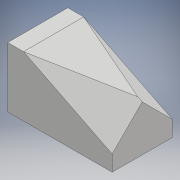
# Autodesk Inventor part: 6431
Saved by Autodesk Inventor 2017 (Build 210142000, 142)
## iProperties
Part Number: 6431
Material: 一般
Document SubType Name: Modeling
Designer: Brian
Density: 1 g/cm^3
Appearance: 預設
Mass: 79.3263 g
Surface Area: 112.179 cm^2
Volume: 79.3263 cm^3
Author: Brian
Autodesk Inventor part; units mm, degrees
ref_plane "YZ Plane" through (0, 0, 0) normal (1, 0, 0) x (0, 1, 0)
ref_plane "XZ Plane" through (0, 0, 0) normal (0, 1, 0) x (-1, 0, 0)
ref_plane "XY Plane" through (0, 0, 0) normal (0, 0, 1) x (1, 0, 0)
sketch "草圖1" plane through (0, 0, 0) normal (0, 1, 0) x (-1, 0, 0)
  line L0 (0, 0) -> (-66, 0)
  line L1 (-66, 0) -> (-66, -38)
  line L2 (-66, -38) -> (0, -38)
  line L3 (0, -38) -> (0, 0)
  dimension "d0" = 66
  dimension "d1" = 38
  constraints: 8 end point, 2 parallel, 1 horizontal, 1 perpendicular
  measures "d0" distance of L1.end L2.end
  measures "d1" distance of L2.end L0.start
extrude "擠出1" add sketch "草圖1" along normal mid plane 38
sketch "草圖2" plane through (0, 19, 0) normal (0, 1, 0) x (1, 0, 0)
  line L0 (0, 0) -> (66, 0) projected
  line L1 (10, 0) -> (66, 8)
  line L2 (66, 0) -> (66, 38) projected
  dimension "d4" = 10
  dimension "d5" = 30
  constraints: 2 end point, 2 point on line
  measures "d4" distance of L0.start L1.start
  measures "d5" distance of L2.end L1.end
extrude "擠出2" cut sketch "草圖2" against normal blind 40
sketch "草圖3" plane through (66, -19, -38) normal (1, 0, 0) x (0, 0, -1)
  line L0 (-30, 18) -> (-10, 38)
  line L1 (0, 38) -> (-38, 38) projected
  line L2 (-30, 38) -> (-30, 0) projected
  point P0 (-38, 19)
  dimension "d8" = 20
  dimension "d9" = 20
  constraints: 2 end point, 2 point on line
  measures "d8" horizontal distance of L0.start L0.end
  measures "d9" horizontal distance of L0.start L0.end
ref_plane "工作平面1" through (10, 19, 0) normal (-0.3333333, -0.6666667, -0.6666667) x (0.8944272, 0, -0.4472136)
sketch "草圖4" plane through (10, 19, 0) normal (-0.3333333, -0.6666667, -0.6666667) x (0.8944272, 0, -0.4472136)
  line L0 (-15.1543, -12.3218) -> (93.717, -12.3218)
  line L1 (93.717, -12.3218) -> (93.717, 28.8166)
  line L2 (93.717, 28.8166) -> (-15.1543, 28.8166)
  line L3 (-15.1543, 28.8166) -> (-15.1543, -12.3218)
  point P0 (-8.9443, 11.1803)
  constraints: 8 end point, 2 parallel, 1 horizontal, 1 perpendicular
extrude "擠出3" cut sketch "草圖4" against normal blind 40
mirror "鏡射1" about plane through (0, 0, 0) normal (0, 1, 0) of "擠出3"
